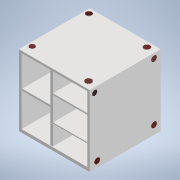
# Autodesk Inventor part: locker 2
Saved by Autodesk Inventor 2022 (Build 260153000, 153)
## iProperties
Created: 2021-07-10
Part Number: locker 2
Material: Generic
Document SubType Name: Modeling
Designer: Hp
Density: 1 g/cm^3
Appearance: Default
Author: Hp
Autodesk Inventor part; units mm, degrees
ref_plane "YZ Plane" through (0, 0, 0) normal (1, 0, 0) x (0, 1, 0)
ref_plane "XZ Plane" through (0, 0, 0) normal (0, 1, 0) x (-1, 0, 0)
ref_plane "XY Plane" through (0, 0, 0) normal (0, 0, 1) x (1, 0, 0)
sketch "Sketch1" plane through (0, 0, 0) normal (0, 0, 1) x (1, 0, 0)
  point P0 (0, 0)
sketch "Sketch2" plane through (0, 0, 0) normal (0, 0, 1) x (1, 0, 0)
  line L0 (-12.8291, 6.9625) -> (-12.8291, -14.6342)
  line L1 (-12.8291, -14.6342) -> (291.9709, -14.6342)
  line L2 (291.9709, -14.6342) -> (291.9709, 290.1658)
  line L3 (291.9709, 290.1658) -> (-12.8291, 290.1658)
  line L4 (-12.8291, 290.1658) -> (-12.8291, -14.6342)
  point P0 (0, 0)
  dimension "d0" = 304.8
  dimension "d1" = 304.8
  dimension "d2" = 304.8
  dimension "d3" = 304.8
  constraints: 10 end point, 3 perpendicular, 1 point on line, 1 vertical
  measures "d0" distance of L0.end L1.end
  measures "d1" distance of L1.end L2.end
  measures "d2" distance of L2.end L3.end
  measures "d3" distance of L3.end L0.end
extrude "Extrusion1" add sketch "Sketch2" along normal blind 304.8
sketch "Sketch3" plane through (0, 0, 304.8) normal (0, 0, 1) x (1, 0, 0)
  line L0 (-1.4082, -1.4082) -> (281.3918, -1.4082)
  line L1 (281.3918, -1.4082) -> (281.3918, 281.3918)
  line L2 (281.3918, 281.3918) -> (-1.4082, 281.3918)
  line L3 (-1.4082, 281.3918) -> (-1.4082, -1.4082)
  line L4 (-1.4082, -1.4082) -> (281.3918, 281.3918) construction
  line L5 (281.3918, -1.4082) -> (-1.4082, 281.3918) construction
  point P0 (0, 0)
  point P1 (139.9918, 139.9918)
  dimension "d8" = 282.8
  dimension "d9" = 282.8
  constraints: 12 end point, 2 midpoint, 2 parallel, 1 horizontal, 1 perpendicular
  measures "d8" distance of L2.end L1.end
  measures "d9" distance of L1.end L0.end
extrude "Extrusion2" cut sketch "Sketch3" against normal blind 302.8
sketch "Sketch4" plane through (0, 0, 2) normal (0, 0, 1) x (1, 0, 0)
  line L0 (-1.4082, 281.3918) -> (281.3918, 281.3918) projected
  line L1 (120.2104, 281.3918) -> (120.2104, -1.4082)
  line L2 (120.2104, -1.4082) -> (130.8619, -1.4082)
  line L3 (281.3918, -1.4082) -> (-1.4082, -1.4082) projected
  line L4 (130.8619, -1.4082) -> (130.8619, 281.3918)
  line L5 (130.8619, 281.3918) -> (120.2104, 281.3918)
  line L6 (281.3918, 281.3918) -> (281.3918, -1.4082) projected
  line L7 (130.8619, 196.2929) -> (281.3918, 196.2929)
  line L8 (281.3918, 196.2929) -> (281.3918, 190.2063)
  line L9 (281.3918, 190.2063) -> (130.8619, 190.2063)
  line L10 (130.8619, 190.2063) -> (130.8619, 196.2929)
  line L11 (130.8619, 88.2557) -> (281.3918, 88.2557)
  line L12 (281.3918, 88.2557) -> (281.3918, 83.6908)
  line L13 (281.3918, 83.6908) -> (130.8619, 83.6908)
  line L14 (130.8619, 83.6908) -> (130.8619, 88.2557)
  line L15 (-1.4082, -1.4082) -> (-1.4082, 281.3918) projected
  line L16 (-1.4082, 139.9918) -> (120.2104, 139.9918)
  line L17 (120.2104, 139.9918) -> (120.2104, 147.6001)
  line L18 (120.2104, 147.6001) -> (-1.4082, 147.6001)
  line L19 (-1.4082, 147.6001) -> (-1.4082, 139.9918)
  point P0 (0, 0)
  point P1 (-1.4082, 147.6001)
  point P2 (120.2104, 139.9918)
  constraints: 32 end point, 7 point on line, 6 parallel, 4 perpendicular, 3 horizontal, 1 midpoint, 1 vertical
extrude "Extrusion3" add sketch "Sketch4" along normal blind 300 contours L0 L4 L2 L1 | L18 L1 L16 L15 | L7 L6 L9 L4 | L11 L6 L13 L4
sketch "Sketch5" plane through (-1.4082, -1.4082, 304.8) normal (1, 0, 0) x (0, 0, -1)
  line L0 (152.8, 241.4577) -> (224.2375, 241.4577) construction
  line L1 (224.2375, 241.4577) -> (224.2375, 189.864) construction
  line L2 (224.2375, 189.864) -> (152.8, 189.864) construction
  line L3 (152.8, 189.864) -> (152.8, 241.4577) construction
  point P0 (304.8, 1.4082)
  constraints: 2 other
sketch "Sketch6" plane through (-1.4082, 281.3918, 304.8) normal (0, -1, 0) x (1, 0, 0)
  line L0 (194.3643, -70.7024) -> (290.2517, -70.7024) construction
  line L1 (290.2517, -70.7024) -> (290.2517, -4.2848) construction
  line L2 (290.2517, -4.2848) -> (194.3643, -4.2848) construction
  line L3 (194.3643, -4.2848) -> (194.3643, -70.7024) construction
  point P0 (1.4082, -304.8)
  constraints: 2 other
decal "Decal1"
decal "Decal2"
sketch "Sketch7" plane through (-12.8291, 290.1658, 0) normal (0, 1, 0) x (1, 0, 0)
  circle A0 centre (19.8924, -23.2079) radius 12.1505
  circle A1 centre (269.1255, -23.2079) radius 13.1175
  circle A2 centre (19.8924, -274.4592) radius 7.0633
  circle A3 centre (269.1255, -274.4592) radius 13.1175
  point P0 (12.8291, 0)
  constraints: 4 centre point
sketch "Sketch8" plane through (-12.8291, 290.1658, 0) normal (0, 1, 0) x (1, 0, 0)
  circle A0 centre (18.8833, -266.3869) radius 10.8677
  point P0 (12.8291, 0)
  constraints: 1 centre point
extrude "Extrusion4" add sketch "Sketch8" along normal blind 2
extrude "Extrusion5" add sketch "Sketch7" along normal blind 2 contours A0 | A1 | A3
sketch "Sketch9" plane through (291.9709, -14.6342, 0) normal (1, 0, 0) x (0, 0, -1)
  circle A0 centre (-285.5587, 286.0663) radius 10.8677
  circle A1 centre (-30.2712, 286.0663) radius 11.9817
  circle A2 centre (-30.2712, 39.8602) radius 12.1505
  circle A3 centre (-274.691, 27.7097) radius 12.1505
  point P0 (0, 14.6342)
  constraints: 4 centre point
extrude "Extrusion6" add sketch "Sketch9" along normal blind 2
sketch "Sketch10" plane through (0, 0, 0) normal (0, 0, -1) x (-1, 0, 0)
  circle A0 centre (-270.423, 270.423) radius 11.7673
  circle A1 centre (-16.1447, 270.423) radius 13.2335
  circle A2 centre (-11.0995, 23.208) radius 11.2814
  circle A3 centre (-270.423, 23.208) radius 11.2814
  point P0 (0, 0)
  constraints: 4 centre point
extrude "Extrusion7" add sketch "Sketch10" along normal blind 2
sketch "Sketch11" plane through (-12.8291, -14.6342, 0) normal (0, -1, 0) x (1, 0, 0)
  point P0 (12.8291, 0)
sketch "Sketch12" plane through (-12.8291, -14.6342, 0) normal (0, -1, 0) x (1, 0, 0)
  circle A0 centre (282.2431, 49.443) radius 13.1563
  circle A1 centre (282.2431, 249.2332) radius 13.1563
  circle A2 centre (53.1907, 36.2867) radius 13.5001
  circle A3 centre (39.6907, 249.2332) radius 13.5001
  point P0 (12.8291, 0)
  constraints: 4 centre point
extrude "Extrusion8" add sketch "Sketch12" along normal blind 2
sketch "Sketch13" plane through (-12.8291, -14.6342, 0) normal (-1, 0, 0) x (0, 0, 1)
  circle A0 centre (30.1663, 40.724) radius 12.2858
  circle A1 centre (30.1663, 264.9329) radius 12.0378
  circle A2 centre (256.0059, 264.9329) radius 14.539
  circle A3 centre (264.9742, 23.6025) radius 13.2296
  point P0 (0, 14.6342)
  constraints: 4 centre point
extrude "Extrusion9" add sketch "Sketch13" along normal blind 2
body "Solid1"
